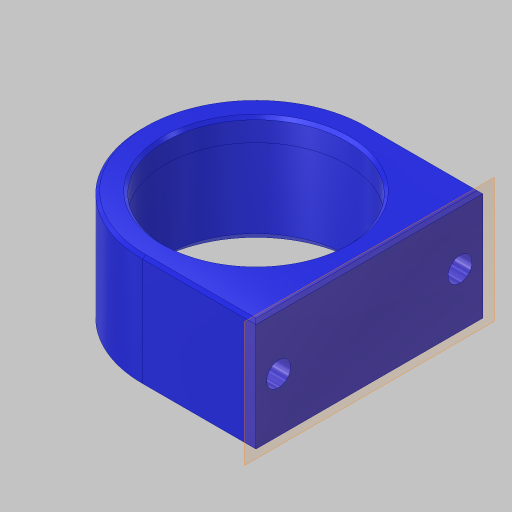
# Autodesk Inventor part: WL-002
Saved by Autodesk Inventor 2023.5 (Build 275446000, 446)
## iProperties
Created: 2025-02-22
Part Number: WL-002
Material: Aluminum 6061
Document SubType Name: Modeling
Designer: slick
Density: 2.7 g/cm^3
Appearance: Blue - Wall Paint - Glossy
Author: slick
Autodesk Inventor part; units mm, degrees
ref_plane "XZ Plane" through (0, 0, 0) normal (0, 1, 0) x (-1, 0, 0)
ref_plane "XY Plane" through (0, 0, 0) normal (0, 0, 1) x (1, 0, 0)
sketch "Sketch1" plane through (0, 0, 0) normal (0, 1, 0) x (-1, 0, 0)
  circle A0 centre (0, 0) radius 25.4
  circle A1 centre (0, 0) radius 31.75
  dimension "d0" = 50.8
  dimension "d1" = 63.5
  constraints: 2 centre point, 2 coincident
  measures "d0" diameter of A0
  measures "d1" diameter of A1
extrude "Extrusion1" add sketch "Sketch1" along normal blind 6.35
sketch "Sketch2" plane through (0, 0, 0) normal (0, -1, 0) x (1, 0, 0)
  circle A0 centre (0, 0) radius 25.654
  circle A1 centre (0, 0) radius 31.75 projected
  dimension "d4" = 51.308
  constraints: 1 centre point, 1 coincident
  measures "d4" diameter of A0
extrude "Extrusion2" add sketch "Sketch2" along normal blind 25.4
chamfer "Chamfer1" distance 3.175 angle 45 1 edges at (-25.654, -25.4, 0)
ref_plane "Work Plane1" through (31.75, 0, 0) normal (1, 0, 0) x (0, 1, 0)
sketch "Sketch5" plane through (31.75, 0, 0) normal (1, 0, 0) x (0, 1, 0)
  line L0 (6.35, 31.75) -> (-25.4, 31.75)
  line L1 (-25.4, -31.75) -> (6.35, -31.75)
  line L2 (6.35, 31.75) -> (-25.4, -31.75) construction
  line L3 (-25.4, 31.75) -> (6.35, -31.75) construction
  line L4 (0, 25.654) -> (0, -25.654) construction
  circle A0 centre (-9.525, 25.4) radius 3.35
  circle A1 centre (-9.525, -25.4) radius 3.35
  line L5 (-9.525, 25.4) -> (-9.525, -25.4) construction
  line L6 (6.35, 31.75) -> (6.35, -31.75)
  line L7 (-25.4, 31.75) -> (-25.4, -31.75)
  point P0 (0, 0)
  point P1 (6.35, 0)
  point P2 (-9.525, 0)
  dimension "d27" = 63.5
  dimension "d28" = 50.8
  dimension "d29" = 6.7
  constraints: 14 end point, 3 midpoint, 2 centre point, 2 horizontal alignment, 2 perpendicular, 1 equal radius, 1 horizontal, 1 parallel, 1 vertical
  measures "d27" distance of L0.end L1.start
  measures "d28" distance of L5.start L5.end
  measures "d29" diameter of A0
extrude "Extrusion4" add sketch "Sketch5" against normal up to surface round surface about axis through (0, 0, 0) along (0, 1, 0) radius 31.75 far side no
chamfer "Chamfer3" distance 0.7937 angle 45 9 edges at (-31.75, 6.35, 0) (15.875, 6.35, 31.75) (15.875, 6.35, -31.75) (25.4, 6.35, 0) (31.75, 6.35, 0) (31.75, -25.4, 0) (15.875, -25.4, -31.75) (-31.75, -25.4, 0) (15.875, -25.4, 31.75)
body "Solid1"
